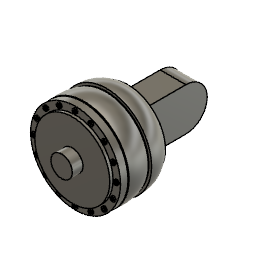
answer (Autodesk Fusion 360 design; units mm, degrees)
part number: 2026-08-05-21-59-05-398
Autodesk Fusion 360 part; units mm, degrees
sketch "Sketch1" plane through (0, 0, 0) normal (0, 1, 0) x (1, 0, 0)
  line L0 (0, 0) -> (-35, 0)
  line L1 (0, 0) -> (0, -20)
  line L2 (0, -20) -> (-42, -20)
  arc A0 (-35, 0) -> (-42, -20) centre (-17.1273, -17.4804) ccw
  dimension "d1" = 35
  dimension "d2" = 20
  dimension "d3" = 42
  dimension "d4" = 25
  constraint coincident L0.start L1.start
  constraint horizontal L0
  constraint perpendicular L0 L1
  constraint perpendicular L1 L2
  measures "d1" distance of L0.start L0.end
  measures "d2" distance of L0.start L1.end
  measures "d3" distance of L1.end L2.end
  measures "d4" radius of A0
revolve "Revolve1" add sketch "Sketch1" angle 360 about axis through (0, 0, 0) along (0, 0, 1)
sketch "Sketch2" plane through (0, 0, 20) normal (0, 0, 1) x (1, 0, 0)
  circle A0 centre (0, 0) radius 42
  circle A1 centre (0, 0) radius 39.5
  dimension "d6" = 79
  constraint concentric A0 A1
  measures "d6" diameter of A1
extrude "Extrude1" add sketch "Sketch2" along normal blind 1 contours A1
sketch "Sketch4" plane through (0, 0, 21) normal (0, 0, 1) x (1, 0, 0)
  circle A0 centre (0, 0) radius 39.5
  constraint coincident A0.centre origin
sketch "Sketch5" plane through (0, 0, 0) normal (0, 1, 0) x (1, 0, 0)
  line L0 (0, -21) -> (0, -41)
  line L1 (0, -41) -> (-42, -41)
  line L2 (0, -21) -> (-40, -21)
  arc A0 (-40, -21) -> (-42, -41) centre (-5.5677, -34.5432) ccw
  point P0 (0, -21)
  dimension "d9" = 20
  dimension "d10" = 42
  dimension "d11" = 40
  dimension "d12" = 37
  constraint vertical L0
  constraint perpendicular L0 L1
  constraint perpendicular L0 L2
  constraint coincident L0 P0
  measures "d9" distance of P0 L0.end
  measures "d10" distance of L0.end L1.end
  measures "d11" distance of P0 L2.end
  measures "d12" radius of A0
revolve "Revolve2" add sketch "Sketch5" angle 360 about axis through (0, 0, 1.75) along (0, 0, 1)
sketch "Sketch6" plane through (0, 0, 41) normal (0, 0, 1) x (1, 0, 0)
  circle A0 centre (0, 0) radius 42
  circle A1 centre (0, 0) radius 41.25
  dimension "d14" = 82.5
  constraint concentric A0 A1
  measures "d14" diameter of A1
extrude "Extrude2" add sketch "Sketch6" along normal blind 1 contours A1
sketch "Sketch7" plane through (0, 0, 42) normal (0, 0, 1) x (1, 0, 0)
  circle A0 centre (0, 0) radius 41.25
  circle A1 centre (0, 0) radius 42
  dimension "d17" = 84
  constraint coincident A0.centre A1.centre
  measures "d17" diameter of A1
extrude "Extrude3" add sketch "Sketch7" along normal blind 7 contours A0 | A1
sketch "Sketch8" plane through (0, 0, 49) normal (0, 0, 1) x (1, 0, 0)
  circle A0 centre (0, 0) radius 42
  circle A1 centre (0, 0) radius 35
  dimension "d20" = 70
  constraint coincident A0.centre A1.centre
  measures "d20" diameter of A1
extrude "Extrude4" add sketch "Sketch8" along normal blind 3 contours A1
sketch "Sketch10" plane through (0, 0, 49) normal (0, 0, 1) x (1, 0, 0)
  circle A0 centre (0, 0) radius 35
  circle A1 centre (0, 0) radius 42
  line L0 (0, 0) -> (35, 0)
  line L1 (42, 0) -> (35, 0)
  circle A2 centre (38.5, 0) radius 3.5
  circle A3 centre (38.5, 0) radius 2.25
  circle A4 centre (38.5, 0) radius 1.5
  dimension "d28" = 4.5
  dimension "d29" = 3
  constraint coincident A0.centre A1.centre
  constraint coincident A0 L0.end
  constraint coincident A1 L1.start
  constraint parallel L0 L1
  constraint coincident L0.end A2
  constraint coincident L1.start A2
  constraint concentric A2 A3
  constraint concentric A2 A4
  measures "d28" diameter of A3
  measures "d29" diameter of A4
extrude "Extrude6" add sketch "Sketch10" along normal blind 1 contours L1 A3 A4 | L1 A3 A4
pattern_circular "C-Pattern1" count 16 over 360 about axis through (0, 0, 52) along (0, 0, 1) of "Extrude6"
sketch "Sketch11" plane through (0, 0, 0) normal (0, 0, -1) x (-1, 0, 0)
  circle A0 centre (0, 0) radius 35
  line L0 (12, 20) -> (-12, 20)
  line L1 (-12, 20) -> (-12, -20)
  line L2 (-12, -20) -> (12, -20)
  line L3 (12, -20) -> (12, 20)
  line L4 (12, 20) -> (-12, -20) construction
  line L5 (-12, 20) -> (12, -20) construction
  dimension "d34" = 40
  dimension "d35" = 24
  constraint horizontal L0
  constraint perpendicular L0 L1
  constraint parallel L0 L2
  constraint parallel L1 L3
  constraint coincident L4 A0.centre
  constraint coincident L5 A0.centre
  constraint coincident A0.centre origin
  measures "d34" distance of L0.start L2.end
  measures "d35" distance of L0.start L0.end
extrude "Extrude7" add sketch "Sketch11" along normal blind 42 contours L0 L1 L2 L3
sketch "Sketch12" plane through (-12, 0, 0) normal (-1, 0, 0) x (0, 0, 1)
  line L0 (0, -20) -> (0, 20)
  line L1 (0, 20) -> (-42, 20)
  line L2 (-42, 20) -> (-42, -20)
  line L3 (-42, -20) -> (0, -20)
  circle A0 centre (-42, 0) radius 20
  dimension "d38" = 40
  constraint midpoint L2 A0.centre
  measures "d38" diameter of A0
extrude "Extrude8" add sketch "Sketch12" against normal blind 24 contours L2 A0 picked at (-48.2058, 2.4356)
sketch "Sketch13" plane through (-12, 0, 0) normal (-1, 0, 0) x (0, 0, 1)
  line L0 (0, -20) -> (0, 20)
  line L1 (0, 20) -> (-42, 20)
  arc A0 (-42, 20) -> (-42, -20) centre (-42, 0) ccw
  line L2 (-42, -20) -> (0, -20)
  circle A1 centre (-40, 0) radius 10
  dimension "d41" = 20
  measures "d41" diameter of A1
extrude "Extrude9" add sketch "Sketch13" along normal blind 10 contours A1
sketch "Sketch14" plane through (0, 0, 52) normal (0, 0, 1) x (1, 0, 0)
  circle A0 centre (0, 0) radius 35
  circle A1 centre (0, 0) radius 10
  dimension "d44" = 20
  constraint coincident A0.centre A1.centre
  measures "d44" diameter of A1
extrude "Extrude10" add sketch "Sketch14" along normal blind 10 contours A1
